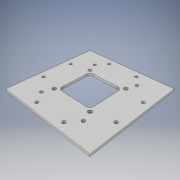
# Autodesk Inventor part: Cougar_Base2
Saved by Autodesk Inventor 2018 (Build 220112000, 112)
## iProperties
Created: 2020-04-13
Part Number: Cougar_Base2
Material: Všeobecné
Document SubType Name: Modeling
Designer: Jozko Mrkvicka
Density: 1 g/cm^3
Appearance: Výchozí
Author: Jozko Mrkvicka
Autodesk Inventor part; units mm, degrees
ref_plane "YZ Plane" through (0, 0, 0) normal (1, 0, 0) x (0, 1, 0)
ref_plane "XZ Plane" through (0, 0, 0) normal (0, 1, 0) x (-1, 0, 0)
ref_plane "XY Plane" through (0, 0, 0) normal (0, 0, 1) x (1, 0, 0)
sketch "Náčrt2" plane through (0, 0, 0) normal (0, 0, 1) x (1, 0, 0)
  line L0 (0, 0) -> (120, 0)
  line L1 (120, 0) -> (120, 120)
  line L2 (120, 120) -> (0, 120)
  line L3 (0, 120) -> (0, 0)
  circle A0 centre (34.5442, 85.4558) radius 2.5
  circle A1 centre (85.4558, 85.4558) radius 2.5
  circle A2 centre (34.5442, 34.5442) radius 2.5
  circle A3 centre (85.4558, 34.5442) radius 2.5
  circle A4 centre (40.5, 111) radius 2
  circle A5 centre (79.5, 111) radius 2
  circle A6 centre (9, 79.5) radius 2
  circle A7 centre (9, 40.5) radius 2
  circle A8 centre (111, 79.5) radius 2
  circle A9 centre (111, 40.5) radius 2
  circle A10 centre (79.5, 9) radius 2
  circle A11 centre (40.5, 9) radius 2
  circle A12 centre (30, 98) radius 2
  circle A13 centre (90, 98) radius 2
  circle A14 centre (90, 22) radius 2
  circle A15 centre (30, 22) radius 2
  line L4 (42.5, 82.5) -> (77.5, 82.5)
  line L5 (82.5, 77.5) -> (82.5, 42.5)
  line L6 (77.5, 37.5) -> (42.5, 37.5)
  line L7 (37.5, 42.5) -> (37.5, 77.5)
  arc A16 (37.5, 42.5) -> (42.5, 37.5) centre (42.5, 42.5) ccw
  arc A17 (77.5, 37.5) -> (82.5, 42.5) centre (77.5, 42.5) ccw
  arc A18 (42.5, 82.5) -> (37.5, 77.5) centre (42.5, 77.5) ccw
  arc A19 (82.5, 77.5) -> (77.5, 82.5) centre (77.5, 77.5) ccw
  point P0 (37.5, 82.5)
  point P1 (82.5, 37.5)
  point P2 (82.5, 82.5)
  point P3 (37.5, 37.5)
  dimension "d18" = 1
  dimension "d26" = 120
  dimension "d27" = 120
  dimension "d28" = 39
  dimension "d29" = 39
  dimension "d30" = 60
  dimension "d31" = 76
  dimension "d32" = 72
  dimension "d35" = 5
  dimension "d36" = 4
  dimension "d37" = 4
  dimension "d42" = 5
  dimension "d43" = 5
  dimension "d44" = 35
  constraints: 20 centre point, 16 end point, 8 point on circle, 8 point on line, 8 tangent, 4 parallel, 2 equal radius, 2 horizontal, 2 perpendicular
  measures "d26" distance of L2.end L1.end
  measures "d27" distance of L1.end L0.end
  measures "d28" distance of A4.centre A5.centre
  measures "d29" distance of A8.centre A9.centre
  measures "d30" distance of A12.centre A13.centre
  measures "d31" distance of A13.centre A14.centre
  measures "d32" distance of A0.centre A3.centre
  measures "d35" diameter of A2
  measures "d36" diameter of A10
  measures "d37" diameter of A15
  measures "d42" radius of A16
  measures "d43" radius of A17
  measures "d44" distance of A17.centre A19.centre
extrude "Vysunutí2" add sketch "Náčrt2" against normal blind 3
